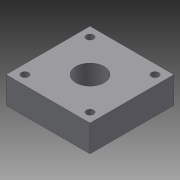
# Autodesk Inventor part: Lead_Screw_Thrust_Bearing_Mount
Saved by Autodesk Inventor 2015 (Build 190159000, 159)
## iProperties
Created: 2014-12-22
Part Number: Lead_Screw_Thrust_Bearing_Mount
Material: Generic
Document SubType Name: Modeling
Designer: Drew
Density: 1 g/cm^3
Appearance: Default
Author: Drew
Autodesk Inventor part; units mm, degrees
ref_plane "YZ Plane" through (0, 0, 0) normal (1, 0, 0) x (0, 1, 0)
ref_plane "XZ Plane" through (0, 0, 0) normal (0, 1, 0) x (-1, 0, 0)
ref_plane "XY Plane" through (0, 0, 0) normal (0, 0, 1) x (1, 0, 0)
sketch "Sketch1" plane through (0, 0, 0) normal (0, 1, 0) x (-1, 0, 0)
  line L0 (-20, -20) -> (20, -20)
  line L1 (20, -20) -> (20, 20)
  line L2 (20, 20) -> (-20, 20)
  line L3 (-20, 20) -> (-20, -20)
  line L4 (-20, -20) -> (20, 20) construction
  line L5 (20, -20) -> (-20, 20) construction
  circle A0 centre (15.5, 15.5) radius 1.75
  line L6 (20, 0) -> (-20, 0)
  line L7 (0, -20) -> (0, 20)
  circle A1 centre (15.5, -15.5) radius 1.75
  circle A2 centre (-15.5, 15.5) radius 1.75
  circle A3 centre (-15.5, -15.5) radius 1.75
  point P0 (0, 0)
  dimension "d3" = 40
  dimension "d4" = 40
  dimension "d5" = 3.5
  dimension "d10" = 31
  dimension "d11" = 31
  constraints: 16 end point, 6 midpoint, 4 centre point, 3 symmetric about line, 2 parallel, 1 horizontal, 1 perpendicular, 1 point on line, 3 other
  measures "d3" distance of L2.end L0.start
  measures "d4" distance of L1.end L2.end
  measures "d5" diameter of A0
  measures "d10" diameter of A2.centre L7
  measures "d11" distance of A3.centre A2.centre
extrude "Extrusion2" add sketch "Sketch1" along normal blind 12.7
sketch "Sketch2" plane through (0, 0, 0) normal (0, -1, 0) x (1, 0, 0)
  circle A0 centre (0, 0) radius 6.75
  dimension "d12" = 13.5
  constraints: 1 centre point, 1 coincident
  measures "d12" diameter of A0
extrude "Extrusion3" cut sketch "Sketch2" against normal through all
body "Solid2"
